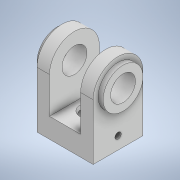
# Autodesk Inventor part: Part3
Saved by Autodesk Inventor 2021 (Build 250183000, 183)
## iProperties
Created: 2022-06-05
Part Number: Part3
Material: Generic
Document SubType Name: Modeling
Designer: Bhargav Malasani
Density: 1 g/cm^3
Appearance: Default
Author: Bhargav Malasani
Autodesk Inventor part; units mm, degrees
ref_plane "YZ Plane" through (0, 0, 0) normal (1, 0, 0) x (0, 1, 0)
ref_plane "XZ Plane" through (0, 0, 0) normal (0, 1, 0) x (-1, 0, 0)
ref_plane "XY Plane" through (0, 0, 0) normal (0, 0, 1) x (1, 0, 0)
sketch "Sketch1" plane through (0, 0, 0) normal (0, 0, 1) x (1, 0, 0)
  line L0 (0, 0) -> (45, 0)
  line L1 (0, 0) -> (0, 65)
  line L2 (0, 65) -> (10, 65)
  line L3 (10, 65) -> (10, 16)
  line L4 (10, 16) -> (22.5, 16)
  line L5 (22.5, 71) -> (22.5, -20)
  line L6 (45, 0) -> (45, 65)
  line L7 (45, 65) -> (35, 65)
  line L8 (35, 65) -> (35, 16)
  line L9 (35, 16) -> (22.5, 16)
  dimension "d1" = 45
  dimension "d2" = 65
  dimension "d3" = 10
  dimension "d4" = 16
  dimension "d5" = 22.5
  constraints: 20 end point, 3 symmetric about line, 2 horizontal, 2 perpendicular, 2 vertical, 1 point on line
  measures "d1" distance of L0.start L0.end
  measures "d2" distance of L0.start L1.end
  measures "d3" distance of L1.end L2.end
  measures "d4" distance between parallel lines of L0 L4
  measures "d5" distance between parallel lines of L5 L1
extrude "Extrusion1" add sketch "Sketch1" along normal mid plane 40
sketch "Sketch2" plane through (0, 0, 20) normal (0, -1, 0) x (1, 0, 0)
  circle A0 centre (22.5, -20) radius 16
  line L0 (0, 0) -> (45, 0) projected
  line L1 (0, -40) -> (0, 0) projected
  point P0 (0, -20)
  dimension "d8" = 32
  dimension "d9" = 20
  dimension "d10" = 22.5
  constraints: 1 centre point
  measures "d8" diameter of A0
  measures "d9" distance from line of L0 A0.centre
  measures "d10" distance from line of L1 A0.centre
extrude "Extrusion2" add sketch "Sketch2" along normal blind 4
fillet "Fillet1" radius 20 4 edges at (5, 65, -20) (5, 65, 20) (40, 65, 20) (40, 65, -20)
sketch "Sketch3" plane through (22.5, -4, 0) normal (0, -1, 0) x (1, 0, 0)
  circle A0 centre (0, 0) radius 16 projected
  circle A1 centre (0, 0) radius 8
  point P0 (-22.5, 0)
  dimension "d14" = 16
  constraints: 1 centre point, 1 coincident
  measures "d14" diameter of A1
extrude "Extrusion3" cut sketch "Sketch3" against normal through all contours A1
sketch "Sketch4" plane through (0, 0, -20) normal (-1, 0, 0) x (0, 0, 1)
  circle A0 centre (20, 45) radius 16
  line L0 (4, -4) -> (36, -4) projected
  line L1 (40, 45) -> (40, 0) projected
  point P0 (20, 0)
  dimension "d17" = 32
  dimension "d18" = 49
  dimension "d19" = 20
  constraints: 1 centre point
  measures "d17" diameter of A0
  measures "d18" distance from line of L0 A0.centre
  measures "d19" distance from line of L1 A0.centre
extrude "Extrusion4" add sketch "Sketch4" along normal blind 4
sketch "Sketch5" plane through (45, 0, 20) normal (1, 0, 0) x (0, 0, -1)
  circle A0 centre (20, 45) radius 16
  line L0 (4, -4) -> (36, -4) projected
  line L1 (0, 0) -> (0, 45) projected
  point P0 (20, 0)
  dimension "d22" = 32
  dimension "d23" = 49
  dimension "d24" = 20
  constraints: 1 centre point
  measures "d22" diameter of A0
  measures "d23" distance from line of L0 A0.centre
  measures "d24" distance from line of L1 A0.centre
extrude "Extrusion5" add sketch "Sketch5" along normal blind 4
sketch "Sketch6" plane through (-4, 45, 0) normal (-1, 0, 0) x (0, 0, 1)
  circle A0 centre (0, 0) radius 16 projected
  circle A1 centre (0, 0) radius 10
  circle A2 centre (0, -35) radius 2.5
  line L0 (-20, -45) -> (20, -45) projected
  line L1 (-20, -45) -> (-20, 0) projected
  point P0 (0, -45)
  dimension "d27" = 20
  dimension "d28" = 5
  dimension "d29" = 10
  dimension "d30" = 20
  constraints: 2 centre point, 1 coincident
  measures "d27" diameter of A1
  measures "d28" diameter of A2
  measures "d29" distance from line of A2.centre L0
  measures "d30" distance from line of L1 A2.centre
extrude "Extrusion6" cut sketch "Sketch6" against normal through all contours A1 | A2
equation "\"d5\" = 0.5 * d1"
body "Solid1"
